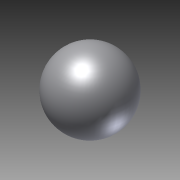
# Autodesk Inventor part: WML5010ZZ Ball
Saved by Autodesk Inventor 2013 SP2 (Build 170200200, 200)
## iProperties
Category: PARTsolutions
Company: KOYO
Created: 2013-06-21
Part Number: WML5010ZZ Ball
Catalog Web Link: www.cadenas.de
Description: Open ball-
Vendor: KOYO
Document SubType Name: Modeling
Designer: PARTuser1
Manufacturer: KOYO
Density: 1 g/cm^3
Material: Generic
PSOL_IDENT_0: {$CADENAS_DATA\23d-libs\koyo\deep_groove_ball_bearings\extra_small_bb_miniature_bb\extra_small_bb_mi
PSOL_IDENT_1: niature_bb\open_ball.prj},175 {VTYP=3D},{NB=WML5010ZZ Ball},{LINA=WML5010ZZ Ball},{NN=Open ball},{DA
PSOL_IDENT_2: TE=21.11.2007 10:19:11},{GEOMDATE=21.11.2007 00:00:00},{VERSION=},{LINEID=1000},{LINESUBID=-1},{WBVA
PSOL_IDENT_3: R=}  {NB=WML5010ZZ Ball},{LINA=WML5010ZZ Ball},{KT=DUMMY},{SRS=BS},{TP=60},{SD=5.0},{D=10},{B=4.0},{
PSOL_IDENT_4: R=0.10},{ORDER=WML5010ZZ},{VERS1=2.0},{ST=2-D},{VERS=2.000},{C=0.43},{C0=0.17},{NG=55000},{NO=0},{SR
PSOL_IDENT_5: =0.20},{DF1=0.0},{BF1=0.0},{BD=1.20},{PCD=7.35},{ID=6.45},{OD=8.25},{GID=6.45},{GOD=8.70},{X1=0.36},
PSOL_IDENT_6: {X2=0.15},{NOB=10}
CNS_NB: WML5010ZZ Ball
CNS_NBSYN: $ORDER. Ball
CNS_LINA: WML5010ZZ Ball
CNS_SRS: BS
CNS_TP: 60
CNS_SD: 5.0
CNS_D: 10
CNS_B: 4.0
CNS_R: 0.10
CNS_ORDER: WML5010ZZ
CNS_VERS1: 2.0
CNS_ST: 2-D
CNS_VERS: 2.000
CNS_C: 0.43
CNS_C0: 0.17
CNS_NG: 55000
CNS_NO: 0
CNS_SR: 0.20
CNS_DF1: 0.0
CNS_BF1: 0.0
CNS_BD: 1.20
CNS_PCD: 7.35
CNS_ID: 6.45
CNS_OD: 8.25
CNS_GID: 6.45
CNS_GOD: 8.70
CNS_X1: 0.36
CNS_X2: 0.15
CNS_NOB: 10
SUPPLIER: KOYO
ARTICLENO: WML5010ZZ Ball
BOMINFO: WML5010ZZ Ball
CREATOR: CADENAS GmbH
Title: WML5010ZZ Ball
Author: Cadenas PARTsolutions
Autodesk Inventor part; units mm, degrees
sketch "Sketch_1" plane through (0, 0, 0) normal (0, 0, 1) x (1, 0, 0)
  line L0 (0.6, 0) -> (-0.6, 0)
  arc A0 (0.6, 0) -> (-0.6, 0) centre (0, 0) ccw
  line L1 (0.6, 0) -> (-0.6, 0)
  constraints: 4 end point, 2 point on circle, 1 centre point
revolve "Revolution1" add sketch "Sketch_1" angle 360 about axis through (0.6, 0, 0) along (1, 0, 0)
ref_plane "ball_XY" through (0, 0, 0) normal (1, 0, 0) x (0, 0, -1)
ref_plane "ball_YZ" through (0, 0, 0) normal (0, 0, -1) x (0, 1, 0)
ref_plane "ball_ZX" through (0, 0, 0) normal (0, 1, 0) x (1, 0, 0)
body "Solid1"
